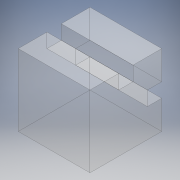
# Autodesk Inventor part: banperparts1
Saved by Autodesk Inventor 2018 (Build 220112000, 112)
## iProperties
Created: 2019-03-06
Part Number: banperparts1
Material: PET プラスチック
Document SubType Name: Modeling
Designer: 西澤　英志
Density: 1.541 g/cm^3
Appearance: ポリカーボネート - クリア
Author: 西澤　英志
Autodesk Inventor part; units mm, degrees
ref_plane "YZ Plane" through (0, 0, 0) normal (1, 0, 0) x (0, 1, 0)
ref_plane "XZ Plane" through (0, 0, 0) normal (0, 1, 0) x (-1, 0, 0)
ref_plane "XY Plane" through (0, 0, 0) normal (0, 0, 1) x (1, 0, 0)
sketch "スケッチ1" plane through (0, 0, 0) normal (1, 0, 0) x (0, 1, 0)
  line L0 (-5, -5) -> (5, -5)
  line L1 (5, -5) -> (5, 5)
  line L2 (5, 5) -> (-5, 5)
  line L3 (-5, 5) -> (-5, -5)
  line L4 (-1, 5) -> (1, 5)
  line L5 (1, 5) -> (1, 3)
  line L6 (1, 3) -> (-1, 3)
  line L7 (-1, 3) -> (-1, 5)
  line L8 (3, -1) -> (5, -1)
  line L9 (5, -1) -> (5, 1)
  line L10 (5, 1) -> (3, 1)
  line L11 (3, 1) -> (3, -1)
  point P0 (0, 0)
  dimension "d0" = 5
  dimension "d1" = 5
  dimension "d2" = 5
  dimension "d3" = 5
  dimension "d4" = 2
  dimension "d5" = 1
  dimension "d6" = 2
  dimension "d7" = 1
  dimension "d8" = 2
  dimension "d9" = 2
  constraints: 24 end point, 6 parallel, 3 horizontal, 3 perpendicular, 2 point on line
  measures "d0" distance from line of point (0, 0) L1
  measures "d1" distance from line of point (0, 0) L3
  measures "d2" distance from line of point (0, 0) L0
  measures "d3" distance from line of point (0, 0) L2
  measures "d4" distance between parallel lines of L7 L5
  measures "d5" distance from line of point (0, 0) L7
  measures "d6" distance between parallel lines of L8 L10
  measures "d7" distance from line of point (0, 0) L8
  measures "d8" distance between parallel lines of L1 L11
  measures "d9" distance between parallel lines of L2 L6
extrude "押し出し1" add sketch "スケッチ1" along normal blind 10 contours L3 L2 L7 L6 L5 L1 L10 L11 L8 L0
